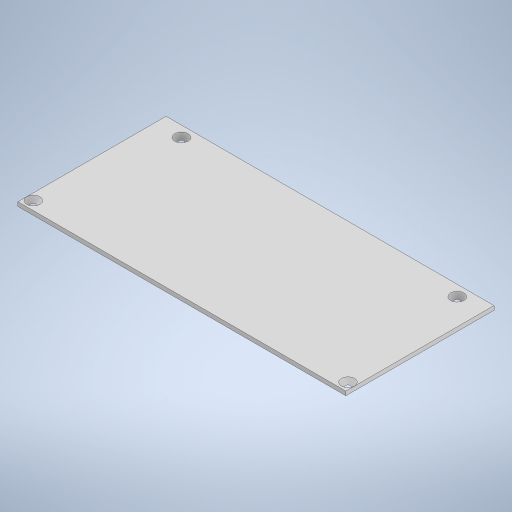
# Autodesk Inventor part: couvercle
Saved by Autodesk Inventor 2024.2 (Build 282272000, 272)
## iProperties
Created: 2024-05-24
Part Number: couvercle
Material: Générique
Document SubType Name: Modeling
Designer: michgae
Density: 1 g/cm^3
Appearance: Par défaut
Author: michgae
Autodesk Inventor part; units mm, degrees
ref_plane "YZ Plane" through (0, 0, 0) normal (1, 0, 0) x (0, 1, 0)
ref_plane "XZ Plane" through (0, 0, 0) normal (0, 1, 0) x (-1, 0, 0)
ref_plane "XY Plane" through (0, 0, 0) normal (0, 0, 1) x (1, 0, 0)
sketch "Esquisse1" plane through (0, 0, 0) normal (0, 1, 0) x (-1, 0, 0)
  line L0 (-80.25, 36.25) -> (80.25, 36.25)
  line L1 (80.25, 36.25) -> (80.25, -36.25)
  line L2 (80.25, -36.25) -> (-80.25, -36.25)
  line L3 (-80.25, -36.25) -> (-80.25, 36.25)
  line L4 (0, -50.75) -> (0, 50.75) projected
  line L5 (112.35, 0) -> (-112.35, 0) projected
  circle A0 centre (77, 32) radius 1.25
  circle A1 centre (-77, 32) radius 1.25
  circle A2 centre (67.5, -31) radius 1.25
  circle A3 centre (-67.5, -31) radius 1.25
  point P0 (0, 0)
  dimension "d0" = 160.5
  dimension "d1" = 72.5
  dimension "d2" = 4.25
  dimension "d3" = 3.25
  dimension "d4" = 2.5
  dimension "d5" = 2.5
  dimension "d6" = 63
  dimension "d7" = 9.5
  constraints: 8 end point, 4 centre point, 2 parallel, 2 symmetric about line, 1 horizontal, 1 perpendicular, 4 other
  measures "d0" distance of L0.start L0.end
  measures "d1" distance of L0.end L1.end
  measures "d2" distance from line of L0 A0.centre
  measures "d3" distance from line of L1 A0.centre
  measures "d4" diameter of A0
  measures "d5" diameter of A2
  measures "d6" vertical distance of A2.centre A0.centre
  measures "d7" horizontal distance of A2.centre A0.centre
extrude "Extrusion1" add sketch "Esquisse1" along normal blind 2
chamfer "Chanfrein1" distance 2 angle 45 4 edges at (-66.25, 2, -31) (-75.75, 2, 32) (78.25, 2, 32) (68.75, 2, -31)
